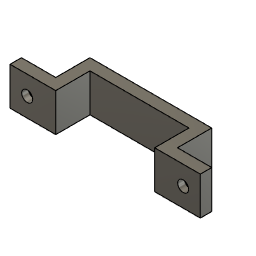
StepperMount v4 (Autodesk Fusion 360 design; units mm, degrees)
Autodesk Fusion 360 part; units mm, degrees
sketch "草图1" plane through (0, 0, 0) normal (0, 1, 0) x (1, 0, 0)
  line L0 (0, 0) -> (12, 0)
  line L1 (12, 0) -> (12, 9)
  line L2 (12, 9) -> (38, 9)
  line L3 (38, 9) -> (38, 0)
  line L4 (38, 0) -> (50, 0)
  line L5 (50, 0) -> (50, 3)
  line L6 (50, 3) -> (41, 3)
  line L7 (41, 3) -> (41, 12)
  line L8 (41, 12) -> (9, 12)
  line L9 (9, 12) -> (9, 3)
  line L10 (9, 3) -> (0, 3)
  line L11 (0, 3) -> (0, 0)
  constraint coincident L0.start L11.end
  constraint horizontal L0
  constraint perpendicular L0 L1
  constraint perpendicular L1 L2
  constraint perpendicular L2 L3
  constraint perpendicular L3 L4
  constraint perpendicular L4 L5
  constraint perpendicular L5 L6
  constraint perpendicular L6 L7
  constraint perpendicular L7 L8
  constraint perpendicular L8 L9
  constraint perpendicular L7 L10
  constraint perpendicular L0 L11
extrude "拉伸1" add sketch "草图1" along normal blind 10
sketch "草图2" plane through (0, 0, -3) normal (0, 0, -1) x (-1, 0, 0)
  line L0 (-9, 0) -> (0, 0)
  line L1 (0, 0) -> (0, 10)
  line L2 (0, 10) -> (-9, 10)
  line L3 (-9, 10) -> (-9, 0)
  circle A0 centre (-4.5, 5) radius 1.5
  dimension "d3" = 3
  measures "d3" diameter of A0
hole "孔1" at (4.5, 5, -3) direction (0, 0, 1) diameter 3 depth 9 tip angle 180
hole "孔2" at (45.5, 5, -3) direction (0, 0, 1) diameter 2.9 depth 10 tip angle 180 countersink diameter 5.3 countersink angle 90
delete_face "删除面1" 1 faces at (4.6494, 6.4925, -1)
move_body "移动1" bodies 1 to x (1, 0, 0) y (0, 1, 0) z (0, 0, 1) at (-25, 0, 0)
hole "孔3" at (-20.5, 5, -3) direction (0, 0, 1) diameter 2.9 depth 10 tip angle 180 countersink diameter 5.3 countersink angle 90
